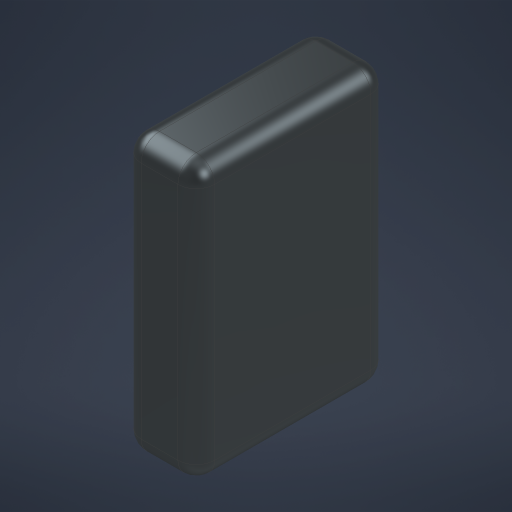
# Autodesk Inventor part: battery
Saved by Autodesk Inventor 2023 (Build 270158000, 158)
## iProperties
Created: 2022-06-23
Part Number: battery
Material: Generic
Document SubType Name: Modeling
Designer: bananenbrot
Density: 1 g/cm^3
Appearance: Default
Author: bananenbrot
Autodesk Inventor part; units mm, degrees
ref_plane "YZ Plane" through (0, 0, 0) normal (1, 0, 0) x (0, 1, 0)
ref_plane "XZ Plane" through (0, 0, 0) normal (0, 1, 0) x (-1, 0, 0)
ref_plane "XY Plane" through (0, 0, 0) normal (0, 0, 1) x (1, 0, 0)
sketch "Sketch1" plane through (0, 0, 0) normal (1, 0, 0) x (0, 1, 0)
  line L0 (49.1461, 21.6404) -> (-40.8539, 21.6404)
  line L1 (-40.8539, 21.6404) -> (-40.8539, -41.3596)
  line L2 (-40.8539, -41.3596) -> (49.1461, -41.3596)
  line L3 (49.1461, -41.3596) -> (49.1461, 21.6404)
  point P0 (0, 0)
  dimension "d0" = 90
  dimension "d1" = 63
  constraints: 8 end point, 2 parallel, 1 horizontal, 1 perpendicular
  measures "d0" distance of L1.end L2.end
  measures "d1" distance of L2.end L0.start
extrude "Extrusion1" add sketch "Sketch1" along normal blind 24
fillet "Fillet1" radius 6 12 edges at (0, 49.1461, -9.8596) (24, 49.1461, -9.8596) (24, -40.8539, -9.8596) (0, -40.8539, -9.8596) (24, 4.1461, 21.6404) (0, 4.1461, 21.6404) (24, 4.1461, -41.3596) (0, 4.1461, -41.3596) (12, -40.8539, -41.3596) (12, -40.8539, 21.6404) (12, 49.1461, -41.3596) (12, 49.1461, 21.6404)
body "Solid1"
